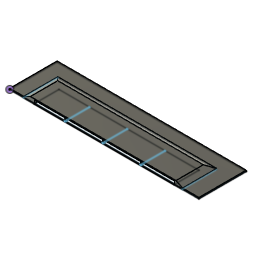
Weichenabdeckung_2Weg_flach v1 (Autodesk Fusion 360 design; units mm, degrees)
Autodesk Fusion 360 part; units mm, degrees
sketch "Skizze2" plane through (0, 0, 0) normal (0, 0, 1) x (1, 0, 0)
  line L0 (0, 0) -> (100, 0)
  line L1 (100, 0) -> (100, 25)
  line L2 (100, 25) -> (0, 25)
  line L3 (0, 25) -> (0, 0)
  line L4 (13, 0) -> (87, 0)
  line L5 (87, 0) -> (87, 13)
  line L6 (87, 13) -> (13, 13)
  line L7 (13, 13) -> (13, 0)
  line L8 (7.3663, 0) -> (91.3663, 0)
  line L9 (91.3663, 0) -> (91.3663, 18)
  line L10 (91.3663, 18) -> (7.3663, 18)
  line L11 (7.3663, 18) -> (7.3663, 0)
  dimension "d1" = 100
  dimension "d2" = 25
  dimension "d3" = 74
  dimension "d4" = 13
  dimension "d5" = 13
  dimension "d6" = 84
  dimension "d7" = 18
  constraint horizontal L0
  constraint vertical L1
  constraint horizontal L2
  constraint vertical L3
  constraint coincident L0.start L3.end
  constraint horizontal L4
  constraint vertical L5
  constraint horizontal L6
  constraint vertical L7
  constraint coincident L0 L4.start
  constraint horizontal L8
  constraint vertical L9
  constraint horizontal L10
  constraint vertical L11
  constraint coincident L0 L8.start
  measures "d1" distance of L0.start L0.end
  measures "d2" distance of L0.start L2.end
  measures "d3" distance of L4.start L4.end
  measures "d4" distance of L4.start L6.end
  measures "d5" distance of L3 L7
  measures "d6" distance of L8.start L8.end
  measures "d7" distance of L8.start L10.end
extrude "Extrusion1" add sketch "Skizze2" along normal blind 0.5 contours L0 L1 L2 L3 L9 L10 L11 makes body 1
extrude "Extrusion2" add sketch "Skizze2" along normal blind 2.2 contours L0 L5 L6 L7 L8 L9 L10 L11 bodies 1
extrude "Extrusion3" add sketch "Skizze2" along normal blind 0.6 from surface at 1.6 contours L0 L4 L5 L6 L7 L8 bodies 1
chamfer "Fase1" distance 3.5 distance2 1.7 1 edges at (91.3663, 9, 2.2) measured on face at (35.3663, 6, 2.2) on bodies 1
chamfer "Fase2" distance 3.5 distance2 1.7 1 edges at (47.6163, 18, 2.2) measured on face at (34.1999, 6, 2.2) on bodies 1
chamfer "Fase3" distance 3.5 distance2 1.7 1 edges at (7.3663, 7.25, 2.2) measured on face at (34.1999, 4.8336, 2.2) on bodies 1
sketch "Skizze3" plane through (0, 0, 0) normal (0, 0, 1) x (1, 0, 0)
  line L0 (49.3454, 12.9531) -> (48.9454, 12.9531)
  line L1 (48.9454, 12.9531) -> (48.9454, 0.1531)
  line L2 (48.9454, 0.1531) -> (49.3454, 0.1531)
  line L3 (49.3454, 0.1531) -> (49.3454, 12.9531)
  line L4 (29.3454, 12.9531) -> (28.9454, 12.9531)
  line L5 (29.3454, 0.1531) -> (29.3454, 12.9531)
  line L6 (28.9454, 12.9531) -> (28.9454, 0.1531)
  line L7 (28.9454, 0.1531) -> (29.3454, 0.1531)
  line L8 (69.3454, 12.9531) -> (68.9454, 12.9531)
  line L9 (69.3454, 0.1531) -> (69.3454, 12.9531)
  line L10 (68.9454, 12.9531) -> (68.9454, 0.1531)
  line L11 (68.9454, 0.1531) -> (69.3454, 0.1531)
  dimension "d21" = 0.4
  dimension "d22" = 12.8
  dimension "d29" = 0
  dimension "d30" = 0
  dimension "d33" = 20
  dimension "d34" = 0
  constraint horizontal L0
  constraint vertical L1
  constraint horizontal L2
  constraint vertical L3
  measures "d21" distance of L0.start L0.end
  measures "d22" distance of L0.start L2.end
extrude "Extrusion4" add sketch "Skizze3" along normal blind 1.6 separate body makes body 2 at (29.3454, 4.4198, 0.5333) makes body 3 at (49.3454, 4.4198, 0.5333) makes body 4 at (69.3454, 4.4198, 0.5333)
